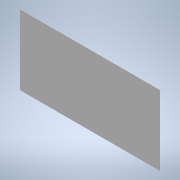
# Autodesk Inventor part: metal jig
Saved by Autodesk Inventor 2020.2 (Build 242310000, 310)
## iProperties
Created: 2020-04-02
Part Number: metal jig
Material: Generic
Document SubType Name: Modeling
Designer: deli
Density: 1 g/cm^3
Appearance: Default
Author: deli
Autodesk Inventor part; units mm, degrees
ref_plane "YZ Plane" through (0, 0, 0) normal (1, 0, 0) x (0, 1, 0)
ref_plane "XZ Plane" through (0, 0, 0) normal (0, 1, 0) x (-1, 0, 0)
ref_plane "XY Plane" through (0, 0, 0) normal (0, 0, 1) x (1, 0, 0)
sketch "Sketch1" plane through (0, 0, 0) normal (0, 0, 1) x (1, 0, 0)
  line L0 (2343.4221, -1116.8175) -> (2343.4221, 102.3825) projected
  line L1 (2343.4221, 102.3825) -> (-94.9779, 102.3825) projected
  line L2 (-94.9779, 102.3825) -> (-94.9779, -1116.8175) projected
  line L3 (-94.9779, -1116.8175) -> (2343.4221, -1116.8175) projected
  point P0 (0, 0)
extrude "Extrusion1" add sketch "Sketch1" along normal blind 3.175
sketch "Sketch2" plane through (0, 0, 3.175) normal (0, 0, 1) x (1, 0, 0)
  line L0 (784.3557, -437.9923) -> (1190.7557, -437.9923) projected
  line L1 (784.3557, -434.8173) -> (1190.7557, -434.8173) projected
  line L2 (784.3557, -511.0173) -> (1190.7557, -511.0173) projected
  line L3 (784.3557, -507.8423) -> (1190.7557, -507.8423) projected
  line L4 (784.3553, -433.5473) -> (1190.7561, -433.5473)
  line L5 (785.9428, -439.2623) -> (1192.3436, -439.2623)
  circle A0 centre (784.3553, -436.4048) radius 2.8575
  point P0 (0, 0)
  dimension "d2" = 1.27
  dimension "d3" = 1.27
  dimension "d4" = 5.715
  dimension "d5" = 5.715
  dimension "d6" = 0
  dimension "d7" = 2.8575
  constraints: 4 end point, 2 parallel, 1 centre point
  measures "d2" distance between parallel lines of L4 L1
  measures "d3" distance between parallel lines of L0 L5
  measures "d4" diameter of A0
  measures "d5" distance between parallel lines of L5 L4
  measures "d6" horizontal distance of L4.start A0.centre
  measures "d7" distance from line of L4 A0.centre
equation "\"d3\" = d2"
equation "\"d4\" = d5"
equation "\"d7\" = 0.5 * d5"
body "Solid1"
